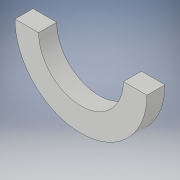
# Autodesk Inventor part: 半円 穴なし
Saved by Autodesk Inventor 2019 (Build 230136000, 136)
## iProperties
Created: 2020-09-25
Part Number: 半円 穴なし
Material: 一般
Document SubType Name: Modeling
Designer: Toshihito
Density: 1 g/cm^3
Appearance: 既定
Author: Toshihito
Autodesk Inventor part; units mm, degrees
ref_plane "YZ Plane" through (0, 0, 0) normal (1, 0, 0) x (0, 1, 0)
ref_plane "XZ Plane" through (0, 0, 0) normal (0, 1, 0) x (-1, 0, 0)
ref_plane "XY Plane" through (0, 0, 0) normal (0, 0, 1) x (1, 0, 0)
sketch "スケッチ1" plane through (0, 0, 0) normal (0, 0, 1) x (1, 0, 0)
  arc A0 (-23.45, 0) -> (23.45, 0) centre (0, 0) ccw
  arc A1 (-36.55, 0) -> (36.55, 0) centre (0, 0) ccw
  line L0 (-48.309, 0) -> (65.7551, 0)
  dimension "d0" = 46.9
  dimension "d1" = 73.1
  constraints: 4 point on circle, 4 point on line, 2 centre point, 2 coincident, 2 end point, 1 horizontal
  measures "d0" diameter of A0
  measures "d1" diameter of A1
extrude "押し出し1" add sketch "スケッチ1" along normal blind 10 contours A0 L0 A1
